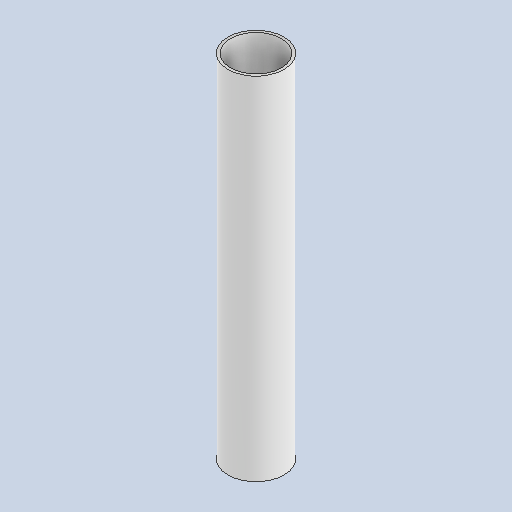
# Autodesk Inventor part: WindTower
Saved by Autodesk Inventor 2024.3 (Build 283343000, 343)
## iProperties
Created: 2024-11-20
Part Number: WindTower
Material: PVC-Rohrsysteme
Document SubType Name: Modeling
Designer: Maximilian Hock
Density: 1.4 g/cm^3
Appearance: Glatt - Weiß
Author: Maximilian Hock
Autodesk Inventor part; units mm, degrees
ref_plane "YZ Plane" through (0, 0, 0) normal (1, 0, 0) x (0, 1, 0)
ref_plane "XZ Plane" through (0, 0, 0) normal (0, 1, 0) x (-1, 0, 0)
ref_plane "XY Plane" through (0, 0, 0) normal (0, 0, 1) x (1, 0, 0)
sketch "Skizze1" plane through (0, 0, 0) normal (0, 0, 1) x (1, 0, 0)
  circle A0 centre (0, 0) radius 16
  circle A1 centre (0, 0) radius 14.5
  dimension "d0" = 29
  dimension "d1" = 32
  constraints: 2 centre point, 2 coincident
  measures "d0" diameter of A1
  measures "d1" diameter of A0
extrude "Extrusion1" add sketch "Skizze1" along normal blind 200
equation "\"d0\" = WindTowerInnerDiameter"
equation "\"d1\" = WindTowerOuterDiameter"
equation "\"d2\" = WindTowerHeight"
equation "\"WindTowerInnerDiameter\" = 29"
equation "\"WindTowerOuterDiameter\" = 32"
equation "\"WindTowerHeight\" = 200"
